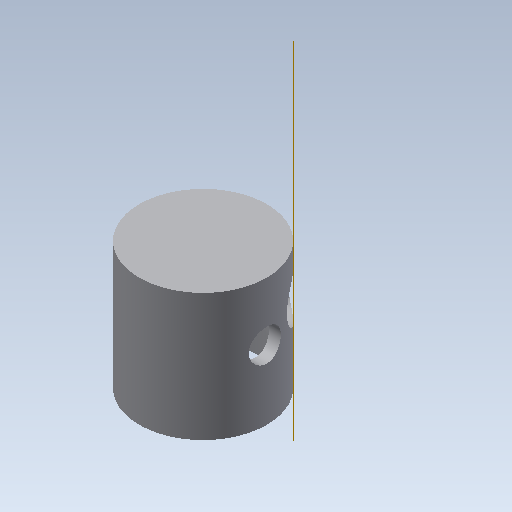
# Autodesk Inventor part: Piston
Saved by Autodesk Inventor 2020 (Build 240152000, 152)
## iProperties
Created: 2012-08-14
Part Number: Piston
Material: Aluminum 6061
Document SubType Name: Modeling
Designer: John
Mass: 1.96844 g
Surface Area: 13.1985 cm^2
Volume: 0.72636 cm^3
Density: 2.71 g/cm^3
Appearance: Aluminum - Flat
Author: John
Autodesk Inventor part; units mm, degrees
ref_plane "YZ Plane" through (0, 0, 0) normal (1, 0, 0) x (0, 1, 0)
ref_plane "XZ Plane" through (0, 0, 0) normal (0, 1, 0) x (-1, 0, 0)
ref_plane "XY Plane" through (0, 0, 0) normal (0, 0, 1) x (1, 0, 0)
sketch "Sketch1" plane through (0, 0, 0) normal (0, 1, 0) x (-1, 0, 0)
  circle A0 centre (0, 0) radius 6.9215
  dimension "d0" = 13.843
  constraints: 1 centre point, 1 coincident
  measures "d0" diameter of A0
extrude "Extrusion1" add sketch "Sketch1" along normal blind 13.843
hole "Hole2" at (0, 0, 0) direction (0, 1, 0) diameter 12.192 depth 3.175
hole "Hole1" at (0, 3.175, 0) direction (0, 1, 0) diameter 11.43 depth 9.144
sketch "Sketch2" plane through (0, 0, 0) normal (1, 0, 0) x (0, 1, 0)
  line L0 (13.843, -6.9215) -> (13.843, 6.9215) projected
  line L1 (13.843, 0) -> (7.493, 0)
  circle A0 centre (7.493, 0) radius 1.7399
  point P0 (0, 0)
  dimension "d21" = 6.35
  dimension "d22" = 3.4798
  constraints: 2 end point, 1 centre point, 1 coincident, 1 midpoint, 1 perpendicular
  measures "d21" distance of L1.start L1.end
  measures "d22" diameter of A0
extrude "Extrusion2" cut sketch "Sketch2" along normal through all both and the other way through all
sketch "Workplane Control Sketch" plane through (0, 13.843, 0) normal (0, 1, 0) x (1, 0, 0)
  circle A0 centre (0, 0) radius 6.9215
  line L0 (0, 0) -> (4.89424, 4.89424)
  line L1 (0, 0) -> (0, 6.9215) construction
  dimension "d25" = 45
  constraints: 4 end point, 2 point on circle, 1 vertical
  measures "d25" angle of L1 L0
ref_plane "Work Plane1" through (4.89424, 13.843, -4.89424) normal (0.7071068, 0, -0.7071068) x (0, 1, 0)
sketch "Sketch4" plane through (4.89424, 13.843, -4.89424) normal (0.7071068, 0, -0.7071068) x (0, 1, 0)
  line L0 (0, 0) -> (-5.08, 0)
  circle A0 centre (-5.08, 0) radius 2.54
  point P0 (-13.843, 0)
  dimension "d26" = 5.08
  dimension "d27" = 5.08
  constraints: 2 end point, 1 centre point, 1 coincident, 1 horizontal
  measures "d26" distance of L0.start L0.end
  measures "d27" diameter of A0
extrude "Extrusion3" cut sketch "Sketch4" against normal up to next
body "Solid1"
